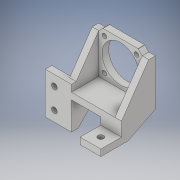
# Autodesk Inventor part: motorBracket
Saved by Autodesk Inventor 2019 (Build 230136000, 136)
## iProperties
Created: 2019-05-07
Part Number: motorBracket
Material: Generic
Document SubType Name: Modeling
Designer: Alex Jones
Density: 1 g/cm^3
Appearance: Default
Author: Alex Jones
Autodesk Inventor part; units mm, degrees
sketch "Sketch1" plane through (0, 0, 0) normal (0, 0, 1) x (1, 0, 0)
  line L0 (-21.15, 16.8267) -> (-21.15, -16.8267) projected
  arc A0 (-21.15, -16.8267) -> (-21.0036, -17.1802) centre (-20.65, -16.8267) ccw projected
  line L1 (-21.0036, -17.1802) -> (-17.1802, -21.0036) projected
  arc A1 (-17.1802, -21.0036) -> (-16.8267, -21.15) centre (-16.8267, -20.65) ccw projected
  line L2 (-16.8267, -21.15) -> (16.8267, -21.15) projected
  arc A2 (16.8267, -21.15) -> (17.1802, -21.0036) centre (16.8267, -20.65) ccw projected
  line L3 (17.1802, -21.0036) -> (21.0036, -17.1802) projected
  arc A3 (21.0036, -17.1802) -> (21.15, -16.8267) centre (20.65, -16.8267) ccw projected
  line L4 (21.15, -16.8267) -> (21.15, 16.8267) projected
  arc A4 (21.15, 16.8267) -> (21.0036, 17.1802) centre (20.65, 16.8267) ccw projected
  line L5 (21.0036, 17.1802) -> (17.1802, 21.0036) projected
  arc A5 (17.1802, 21.0036) -> (16.8267, 21.15) centre (16.8267, 20.65) ccw projected
  line L6 (16.8267, 21.15) -> (-16.8267, 21.15) projected
  arc A6 (-16.8267, 21.15) -> (-17.1802, 21.0036) centre (-16.8267, 20.65) ccw projected
  line L7 (-17.1802, 21.0036) -> (-21.0036, 17.1802) projected
  arc A7 (-21.0036, 17.1802) -> (-21.15, 16.8267) centre (-20.65, 16.8267) ccw projected
  circle A8 centre (-15.5, -15.5) radius 1.75 projected
  circle A9 centre (-15.5, 15.5) radius 1.75 projected
  circle A10 centre (15.5, 15.5) radius 1.75 projected
  circle A11 centre (15.5, -15.5) radius 1.75 projected
  circle A12 centre (0, 0) radius 17 projected
  circle A13 centre (15.5, 15.5) radius 2.2144
  circle A14 centre (15.5, -15.5) radius 2.2144
  circle A15 centre (-15.5, -15.5) radius 2.2144
  circle A16 centre (-15.5, 15.5) radius 2.2144
  circle A17 centre (0, 0) radius 17.7962
  constraints: 5 centre point, 3 equal radius
extrude "Extrusion1" add sketch "Sketch1" along normal blind 6.35 contours A7 L7 A6 L6 A5 L5 A4 L4 A3 L3 A2 L2 A1 L1 A0 L0
sketch "Sketch2" plane through (-16.8267, -21.15, 0) normal (0, -1, 0) x (1, 0, 0)
  line L0 (0, 0) -> (33.6533, 0) projected
  line L1 (33.6533, 0) -> (33.6533, 6.35) projected
  line L2 (0, 6.35) -> (33.6533, 6.35) projected
  line L3 (0, 0) -> (0, 6.35) projected
  line L4 (-10.6733, 32.7) -> (65.5267, 32.7) projected
  line L5 (65.5267, 33.95) -> (-10.6733, 33.95) projected
  line L6 (65.5267, 33.95) -> (65.5267, 39.1) projected
  line L7 (65.5267, 39.1) -> (-10.6733, 39.1) projected
  line L8 (-10.6733, 33.95) -> (-10.6733, 39.1) projected
  line L9 (0, 0) -> (33.6533, 0)
  line L10 (33.6533, 0) -> (33.6533, 32.7)
  line L11 (33.6533, 32.7) -> (0, 32.7)
  line L12 (0, 32.7) -> (0, 0)
  line L13 (-4.1769, 0) -> (-0.3536, 0) projected
  line L14 (-0.3536, 0) -> (-0.3536, 6.35) projected
  line L15 (-4.1769, 6.35) -> (-0.3536, 6.35) projected
  line L16 (-4.1769, 0) -> (-4.1769, 6.35) projected
  line L17 (34.0069, 0) -> (37.8302, 0) projected
  line L18 (37.8302, 0) -> (37.8302, 6.35) projected
  line L19 (34.0069, 6.35) -> (37.8302, 6.35) projected
  line L20 (34.0069, 0) -> (34.0069, 6.35) projected
  line L21 (-4.1769, 0) -> (37.8302, 0)
  line L22 (37.8302, 0) -> (37.8302, 32.7)
  line L23 (37.8302, 32.7) -> (-4.1769, 32.7)
  line L24 (-4.1769, 32.7) -> (-4.1769, 0)
  point P0 (16.8267, 0)
  constraints: 16 end point, 4 parallel, 2 horizontal, 2 perpendicular, 2 point on line
extrude "Extrusion2" add sketch "Sketch2" along normal blind 6.35 contours L3 L2 L1 L0 | L21 L14 L15 L24 L4 L12 L3 | L1 L10 L4 L22 L19 L20 L21 | L12 L4 L10 L2 | L13 L16 L15 L14 | L20 L19 L18 L17
ref_plane "Work Plane1" through (0, -21.15, 0) normal (-1, 0, 0) x (0, 0, 1)
sketch "Sketch4" plane through (-21.0036, -21.15, 0) normal (-1, 0, 0) x (0, 0, 1)
  line L0 (0, 37.9767) -> (0, 4.3233) projected
  line L1 (0, 4.3233) -> (6.35, 4.3233) projected
  line L2 (6.35, 37.9767) -> (6.35, 4.3233) projected
  line L3 (0, 37.9767) -> (6.35, 37.9767) projected
  line L4 (32.7, 0) -> (0, 0) projected
  line L5 (0, 0) -> (0, -6.35) projected
  line L6 (32.7, -6.35) -> (0, -6.35) projected
  line L7 (32.7, 0) -> (32.7, -6.35) projected
  line L8 (6.35, 37.9767) -> (6.35, 4.3233) projected
  line L9 (32.7, 0) -> (32.7, -6.35) projected
  line L10 (0, 0.1464) -> (6.35, 0.1464) projected
  line L11 (0, 38.3302) -> (6.35, 38.3302) projected
  line L12 (0, 38.3302) -> (6.35, 38.3302)
  line L13 (6.35, 38.9462) -> (6.35, 3.3538) projected
  line L14 (6.35, 38.3302) -> (32.7, 0)
  line L15 (0, 0) -> (0, -6.35) projected
  line L16 (32.7, 0) -> (0, 0)
  line L17 (0, 0) -> (0, 38.3302)
  point P0 (0, 21.15)
  constraints: 8 end point, 2 perpendicular, 1 point on line
extrude "Extrusion3" add sketch "Sketch4" along normal blind 6.35
mirror "Mirror1" about plane through (0, -21.15, 0) normal (-1, 0, 0) of "Extrusion3"
sketch "Sketch5" plane through (-16.8267, -27.5, 0) normal (0, -1, 0) x (1, 0, 0)
  line L0 (2.5767, 45.45) -> (8.0767, 45.45) projected
  arc A0 (8.0767, 39.95) -> (8.0767, 45.45) centre (8.0767, 42.7) ccw projected
  line L1 (8.0767, 39.95) -> (2.5767, 39.95) projected
  arc A1 (2.5767, 45.45) -> (2.5767, 39.95) centre (2.5767, 42.7) ccw projected
  line L2 (17.3267, 50.7) -> (-6.6733, 50.7) projected
  line L3 (-6.6733, 50.7) -> (-6.6733, 34.7) projected
  line L4 (-6.6733, 34.7) -> (17.3267, 34.7) projected
  line L5 (17.3267, 34.7) -> (17.3267, 50.7) projected
  line L6 (-10.5269, 32.7) -> (44.1802, 32.7) projected
  line L7 (-10.5269, 0) -> (-10.5269, 32.7) projected
  line L8 (44.1802, 0) -> (-10.5269, 0) projected
  line L9 (44.1802, 0) -> (44.1802, 32.7) projected
  line L10 (37.8302, 32.7) -> (44.1802, 32.7) projected
  line L11 (44.1802, 32.7) -> (24.1802, 32.7)
  line L12 (24.1802, 32.7) -> (24.1802, 26.35)
  line L13 (24.1802, 26.35) -> (44.1802, 26.35)
  line L14 (44.1802, 26.35) -> (44.1802, 32.7)
  point P0 (16.8267, 0)
  dimension "d6" = 20
  dimension "d7" = 6.35
  constraints: 8 end point, 2 parallel, 1 horizontal, 1 perpendicular
  measures "d6" distance of L12.end L13.end
  measures "d7" distance of L11.end L12.end
ref_plane "Work Plane2" through (-27.5, -34.5, 33.95) normal (0, -1, 0) x (1, 0, 0)
extrude "Extrusion4" add sketch "Sketch5" along normal up to surface (7 mm away) contours L6 L9 L13 L12
sketch "Sketch6" plane through (7.3536, -34.5, 32.7) normal (0, -1, 0) x (1, 0, 0)
  line L0 (20, 0) -> (20, -6.35) projected
  line L1 (0, 0) -> (20, 0) projected
  line L2 (0, -6.35) -> (0, 0) projected
  line L3 (20, -6.35) -> (0, -6.35) projected
  point P0 (-7.3536, -32.7)
extrude "Extrusion5" add sketch "Sketch6" along normal blind 6.35
sketch "Sketch7" plane through (-27.3536, -21.15, 32.7) normal (0, 0, 1) x (1, 0, 0)
  line L0 (34.7071, -6.35) -> (34.7071, -19.7) projected
  line L1 (54.7071, 0) -> (54.7071, -19.7) projected
  line L2 (34.7071, -19.7) -> (54.7071, -19.7)
  line L3 (54.7071, -19.7) -> (54.7071, -13.35)
  line L4 (54.7071, -13.35) -> (34.7071, -13.35)
  line L5 (34.7071, -13.35) -> (34.7071, -19.7)
  point P0 (27.3536, 21.15)
  dimension "d12" = 6.35
  constraints: 8 end point, 2 parallel, 1 horizontal, 1 perpendicular, 1 point on line
  measures "d12" distance between parallel lines of L2 L4
extrude "Extrusion6" add sketch "Sketch7" along normal blind 20
sketch "Sketch8" plane through (7.3536, -40.85, 32.7) normal (0, -1, 0) x (1, 0, 0)
  line L0 (20, 20) -> (0, 20) projected
  line L1 (20, -6.35) -> (20, 20) projected
  line L2 (0, 20) -> (20, 20)
  line L3 (20, 20) -> (20, 0)
  line L4 (20, 0) -> (0, 0)
  line L5 (0, 0) -> (0, 20)
  circle A0 centre (10, 10) radius 2.75
  point P0 (-7.3536, -32.7)
  dimension "d15" = 20
  dimension "d16" = 5.5
  constraints: 8 end point, 2 parallel, 1 centre point, 1 horizontal, 1 perpendicular, 1 point on line
  measures "d15" distance between parallel lines of L0 L4
  measures "d16" diameter of A0
extrude "Extrusion7" cut sketch "Sketch8" against normal blind 20 contours A0
ref_plane "Work Plane3" through (-33.9, -14.5, 32.7) normal (0, 0, -1) x (0, 1, 0)
sketch "Sketch9" plane through (-33.9, -14.5, 32.7) normal (0, 0, -1) x (0, 1, 0)
  line L0 (0, -12.35) -> (-1000, -12.35) projected
  line L1 (0, -12.35) -> (0, -7.2) projected
  line L2 (0, -7.2) -> (-1000, -7.2) construction
  line L3 (-1000, -12.35) -> (-1000, -7.2) projected
  line L4 (-1000, 5.15) -> (0, 5.15) construction
  line L5 (-1000, 0) -> (-1000, 5.15) projected
  line L6 (0, 0) -> (-1000, 0) construction
  line L7 (0, 0) -> (0, 5.15) projected
  line L8 (0, 5.15) -> (-40, 5.15) construction
  line L9 (-40, 5.15) -> (-40, -12.35)
  line L10 (-40, -12.35) -> (0, -12.35)
  line L11 (0, -12.35) -> (0, 5.15)
  line L12 (-6.5036, 51.0802) -> (-2.6802, 54.9036) projected
  arc A0 (-6.5036, 51.0802) -> (-6.65, 50.7267) centre (-6.15, 50.7267) ccw projected
  line L13 (-6.65, 50.7267) -> (-6.65, 54.9036) projected
  line L14 (-2.6802, 54.9036) -> (-6.65, 54.9036) projected
  line L15 (31.6802, 54.9036) -> (31.6802, 61.2536) projected
  line L16 (31.6802, 61.2536) -> (-13, 61.2536) projected
  line L17 (-13, 61.2536) -> (-13, 6.5464) projected
  line L18 (31.6802, 6.5464) -> (-13, 6.5464) projected
  line L19 (31.6802, 12.8964) -> (31.6802, 6.5464) projected
  line L20 (35.5036, 16.7198) -> (31.6802, 12.8964) projected
  arc A1 (35.5036, 16.7198) -> (35.65, 17.0733) centre (35.15, 17.0733) ccw projected
  line L21 (35.65, 50.7267) -> (35.65, 17.0733) projected
  arc A2 (35.65, 50.7267) -> (35.5036, 51.0802) centre (35.15, 50.7267) ccw projected
  line L22 (31.6802, 54.9036) -> (35.5036, 51.0802) projected
  line L23 (-6.65, 12.8964) -> (-6.65, 17.0733) projected
  arc A3 (-6.65, 17.0733) -> (-6.5036, 16.7198) centre (-6.15, 17.0733) ccw projected
  line L24 (-2.6802, 12.8964) -> (-6.5036, 16.7198) projected
  line L25 (-2.6802, 12.8964) -> (-6.65, 12.8964) projected
  circle A4 centre (14.5, 33.9) radius 17.7962 projected
  circle A5 centre (30, 18.4) radius 2.2144 projected
  circle A6 centre (-1, 18.4) radius 2.2144 projected
  circle A7 centre (-1, 49.4) radius 2.2144 projected
  circle A8 centre (30, 49.4) radius 2.2144 projected
  line L26 (0, 5.15) -> (-40, 5.15) construction
  line L27 (-40, 5.15) -> (-40, 6.5464)
  line L28 (-40, 6.5464) -> (0, 6.5464)
  line L29 (0, 6.5464) -> (0, 5.15)
  line L30 (-20, -3.6) -> (-40, -3.6) construction
  line L31 (-20, -12.35) -> (-20, 6.5464) construction
  line L32 (-20, -3.6) -> (0, -3.6) construction
  circle A9 centre (-10, -3.6) radius 2.75
  circle A10 centre (-30, -3.6) radius 2.75
  line L33 (0, -12.35) -> (-40, -12.35)
  line L34 (-40, -12.35) -> (-40, 6.5464)
  line L35 (-40, 6.5464) -> (0, 6.5464)
  line L36 (0, 6.5464) -> (0, -12.35)
  dimension "d19" = 40
  dimension "d20" = 5.5
  constraints: 30 end point, 6 midpoint, 6 parallel, 3 horizontal, 3 perpendicular, 2 centre point, 2 point on line, 1 equal radius
  measures "d19" distance between parallel lines of L11 L9
  measures "d20" diameter of A9
extrude "Extrusion8" add sketch "Sketch9" along normal blind 6.35 contours L0 L9 L27 L28 L18 L29 L7 L11 L1
sketch "Sketch10" plane through (-27.3536, -54.5, 32.7) normal (1, 0, 0) x (0, 0, -1)
  line L0 (-1.6, 40) -> (-1.6, -960) projected
  line L1 (6.35, 27) -> (0, 27) projected
  line L2 (0, 27) -> (0, 0) projected
  line L3 (0, 0) -> (6.35, 0) projected
  line L4 (6.35, 27) -> (6.35, 0) projected
  point P0 (32.7, 54.5)
extrude "Extrusion9" add sketch "Sketch10" along normal blind 6.35
sketch "Sketch11" plane through (-21.0036, -54.5, 32.7) normal (1, 0, 0) x (0, 0, -1)
  line L0 (0, 27) -> (6.35, 27) projected
  line L1 (0, 27) -> (0, 0) projected
  line L2 (0, 0) -> (6.35, 0) projected
  line L3 (6.35, 0) -> (6.35, 27) projected
  line L4 (32.7, 27) -> (6.35, 27) projected
  line L5 (0, 0) -> (6.35, 0) projected
  line L6 (32.7, 27) -> (6.35, 0)
  line L7 (6.35, 27) -> (6.35, 13.65) projected
  line L8 (6.35, 0) -> (6.35, 27)
  line L9 (32.7, 71.6802) -> (32.7, 27) projected
  line L10 (6.35, 27) -> (32.7, 27)
  point P0 (32.7, 54.5)
  constraints: 6 end point, 1 collinear, 1 perpendicular
extrude "Extrusion10" add sketch "Sketch11" against normal blind 6.35 contours L4 L6 L3
sketch "Sketch12" plane through (-27.3536, -21.15, 32.7) normal (1, 0, 0) x (0, 0, -1)
  line L0 (0, 0) -> (4.5715, 6.65) projected
  line L1 (0, 6.65) -> (4.5715, 6.65) projected
  line L2 (0, 6.65) -> (0, 0) projected
  point P0 (32.7, 21.15)
extrude "Extrusion11" add sketch "Sketch12" along normal up to surface (6.35 mm away)
sketch "Sketch13" plane through (27.3536, -27.5, 0) normal (1, 0, 0) x (0, 0, -1)
  line L0 (0, 44.6802) -> (0, 0) projected
  line L1 (-6.35, 44.6802) -> (0, 44.6802) projected
  line L2 (-32.7, 6.35) -> (-6.35, 44.6802) projected
  line L3 (-32.7, 6.35) -> (-32.7, -7) projected
  line L4 (-32.7, -7) -> (-52.7, -7) projected
  line L5 (-52.7, -13.35) -> (-52.7, -7) projected
  line L6 (-26.35, -13.35) -> (-52.7, -13.35) projected
  line L7 (-26.35, 0) -> (-26.35, -13.35) projected
  line L8 (0, 0) -> (-26.35, 0) projected
  line L9 (-26.35, -13.35) -> (0, 0)
  line L10 (-26.35, 0) -> (-26.35, -13.35)
  line L11 (-26.35, 13) -> (-26.35, -27) projected
  line L12 (-32.7, 0) -> (0, 0) projected
  line L13 (-26.35, 0) -> (0, 0)
  point P0 (0, 27.5)
  constraints: 6 end point, 1 collinear, 1 horizontal
extrude "Extrusion12" add sketch "Sketch13" against normal up to surface (20 mm away) contours L9 L7 L8
sketch "Sketch14" plane through (0, 0, 0) normal (0, 0, -1) x (-1, 0, 0)
  line L0 (-17.1802, -21.0036) -> (-21.0036, -17.1802) projected
  arc A0 (-17.1802, -21.0036) -> (-16.8267, -21.15) centre (-16.8267, -20.65) ccw projected
  line L1 (-16.8267, -21.15) -> (-21.0036, -21.15) projected
  line L2 (-21.0036, -17.1802) -> (-21.0036, -21.15) projected
  line L3 (-21.0036, 17.1802) -> (-27.3536, 17.1802) projected
  line L4 (-27.3536, 17.1802) -> (-27.3536, -27.5) projected
  line L5 (-27.3536, -27.5) -> (-7.3536, -27.5) projected
  line L6 (-7.3536, -27.5) -> (21.0036, -27.5) projected
  line L7 (21.0036, -27.5) -> (27.3536, -27.5) projected
  line L8 (27.3536, 17.1802) -> (27.3536, -27.5) projected
  line L9 (21.0036, 17.1802) -> (27.3536, 17.1802) projected
  line L10 (17.1802, 21.0036) -> (21.0036, 17.1802) projected
  arc A1 (17.1802, 21.0036) -> (16.8267, 21.15) centre (16.8267, 20.65) ccw projected
  line L11 (-16.8267, 21.15) -> (16.8267, 21.15) projected
  arc A2 (-16.8267, 21.15) -> (-17.1802, 21.0036) centre (-16.8267, 20.65) ccw projected
  line L12 (-21.0036, 17.1802) -> (-17.1802, 21.0036) projected
  line L13 (21.0036, -21.15) -> (16.8267, -21.15) projected
  arc A3 (16.8267, -21.15) -> (17.1802, -21.0036) centre (16.8267, -20.65) ccw projected
  line L14 (21.0036, -17.1802) -> (17.1802, -21.0036) projected
  line L15 (21.0036, -17.1802) -> (21.0036, -21.15) projected
  circle A4 centre (0, 0) radius 17.7962 projected
  circle A5 centre (15.5, 15.5) radius 2.2144 projected
  circle A6 centre (15.5, -15.5) radius 2.2144 projected
  circle A7 centre (-15.5, -15.5) radius 2.2144 projected
  circle A8 centre (-15.5, 15.5) radius 2.2144 projected
extrude "Extrusion13" add sketch "Sketch14" against normal up to surface (6.35 mm away) contours A0 L1 L2 L0 | L13 A3 L14 L15
body "Solid1"
